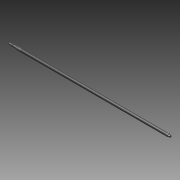
# Autodesk Inventor part: BNT 2010-2.61000-J1K Shaft
Saved by Autodesk Inventor 2016 (Build 200138000, 138)
## iProperties
Category: PARTsolutions
Company: THK
Created: 2017-05-30
Part Number: BNT 2010-2.61000-J1K Shaft
Catalog Web Link: www.cadenas.de
Description: BNT Shaft-
Vendor: THK
Document SubType Name: Modeling
Designer: psAdmin
Manufacturer: THK
Mass: 354.556 g
Surface Area: 729.515 cm^2
Volume: 354.556 cm^3
Density: 1 g/cm^3
Material: Generic
Appearance: PSOLRGB-192-192-192
PSOL_IDENT_0: {$CADENAS_DATA\23d-libs\thk\fed_screw\ball_screw\ball_screw\standard_lead_rbs\bnt\bnt_shaft.prj},206
PSOL_IDENT_1: {VTYP=3D},{NB=BNT 2010-2.61000-J1K Shaft},{LINA=BNT 2010-2.61000-J1K Shaft},{NN=BNT Shaft},{DATE=16
PSOL_IDENT_2: .05.2017 06:09:49},{GEOMDATE=28.04.2017 11:55:02},{VERSION=},{LINEID=520},{LINESUBID=-1},{WBVAR=ST,F
PSOL_IDENT_3: S,SS}  {NB=BNT 2010-2.61000-J1K Shaft},{LINA=BNT 2010-2.61000-J1K Shaft},{KT=DUMMY},{MN=BNT 2010-2.6
PSOL_IDENT_4: },{ST=1000},{FS=-J1},{SS=K},{OL=1166},{EL=2092},{L=58},{R1=11.300},{R2=11.300},{T1=2.500},{T2=2.500}
PSOL_IDENT_5: ,{P3=16.000},{P4=16.000},{B3=14.300},{B4=14.300},{G2=4.000},{G3=1.150},{G4=1.150},{F3=10.150},{F4=10
PSOL_IDENT_6: .150},{A3=15.000},{A4=15.000},{G1=4.000},{S1=12.000},{S2=13.000},{A1=15.000},{A2=15.000},{B1=12.000}
PSOL_IDENT_7: ,{B2=12.000},{J1=16.000},{SD=20},{J2=16.000},{M1=15.000},{M2=15.000},{P11=1.000},{P2=1.000},{P1=2.50
PSOL_IDENT_8: 0},{FSX='','None','-H1','Type_H1','-H2','Type_H2','-H3','Type_H3','-J1','Type_J1','-J2','Type_J2','-
PSOL_IDENT_9: J3','Type_J3'},{E3=13},{E4=13},{F1=20},{E1=40},{N1=6},{H1=9},{F2=20},{E2=49},{N2=6},{H2=9},{STX=2034
PSOL_IDENT_10: },{FSX1=75},{SSX1=13},{VERMN=1},{VERK=1}
NN: BNT Shaft
NB: BNT 2010-2.61000-J1K Shaft
NBSYN: $MN.$ST.$FS.$SS. Shaft
LINA: BNT 2010-2.61000-J1K Shaft
MN: BNT 2010-2.6
ST: 1000
FS: Type_J1
SS: Type_K
EL: 2092
L: 58
R1: 11.300
R2: 11.300
T1: 2.500
T2: 2.500
P3: 16.000
P4: 16.000
B3: 14.300
B4: 14.300
G2: 4.000
G3: 1.150
G4: 1.150
F3: 10.150
F4: 10.150
A3: 15.000
A4: 15.000
G1: 4.000
S1: 12.000
S2: 13.000
A1: 15.000
A2: 15.000
B1: 12.000
B2: 12.000
J1: 16.000
SD: 20
J2: 16.000
M1: 15.000
M2: 15.000
P11: 1.000
P2: 1.000
P1: 2.500
FSX: '','None','-H1','Type_H1','-H2','Type_H2','-H3','Type_H3','-J1','Type_J1','-J2','Type_J2','-J3','Type_J3'
E3: 13
E4: 13
F1: 20
E1: 40
N1: 6
H1: 9
F2: 20
E2: 49
N2: 6
H2: 9
VERMN: 1
SUPPLIER: THK
ARTICLENO: BNT 2010-2.61000-J1K Shaft
BOMINFO: BNT 2010-2.61000-J1K Shaft
CREATOR: CADENAS GmbH
Title: BNT 2010-2.61000-J1K Shaft
Author: Cadenas PARTsolutions
Autodesk Inventor part; units mm, degrees
ref_plane "YZ Plane" through (0, 0, 0) normal (1, 0, 0) x (0, 1, 0)
ref_plane "XZ Plane" through (0, 0, 0) normal (0, 1, 0) x (-1, 0, 0)
ref_plane "XY Plane" through (0, 0, 0) normal (0, 0, 1) x (1, 0, 0)
sketch "Sketch_1" plane through (0, 0, 0) normal (0, 0, 1) x (1, 0, 0)
  line L0 (1068, 0) -> (10, 0)
  line L1 (10, 0) -> (10, 10)
  line L2 (10, 10) -> (1068, 10)
  line L3 (1068, 10) -> (1068, 0)
  line L4 (1068, 0) -> (10, 0)
  constraints: 10 end point
revolve "Revolution1" add sketch "Sketch_1" angle 360 about axis through (1068, 0, 0) along (1, 0, 0)
thread "Thread1" size "M20x2.5" class "6g" standard "ISO Metric profile" full length
sketch "Sketch_10" plane through (0, 0, 0) normal (0, 1, 0) x (-1, 0, 0)
  line L0 (-10, 0) -> (75, 0)
  line L1 (75, 0) -> (75, -5.3333)
  line L2 (75, -5.3333) -> (74.3333, -6)
  line L3 (74.3333, -6) -> (55, -6)
  line L4 (55, -6) -> (55, -6.8865)
  line L5 (55, -6.8865) -> (54.3865, -7.5)
  line L6 (54.3865, -7.5) -> (15, -7.5)
  line L7 (15, -7.5) -> (15, -9)
  line L8 (15, -9) -> (14, -10)
  line L9 (14, -10) -> (-9.8, -10)
  line L10 (-9.8, -10) -> (-9.8, -8)
  line L11 (-9.8, -8) -> (-10, -8)
  line L12 (-10, -8) -> (-10, 0)
  line L13 (-10, 0) -> (75, 0)
  constraints: 28 end point
revolve "Revolution2" add sketch "Sketch_10" angle 360 about axis through (10, 0, 0) along (1, 0, 0)
thread "Thread2" size "M15x1" class "6g" standard "ISO Metric profile" length 11.3865
sketch "Sketch_11" plane through (0, 0, 8) normal (0, 0, 1) x (1, 0, 0)
  line L0 (-9, -10) -> (0, -10)
  line L1 (0, -10) -> (0, 10)
  line L2 (0, 10) -> (-9, 10)
  line L3 (-9, 10) -> (-9, -10)
  constraints: 8 end point
extrude "Extrusion1" cut sketch "Sketch_11" along normal blind 4
sketch "Sketch_12" plane through (0, 0, -8) normal (0, 0, 1) x (1, 0, 0)
  line L0 (-9, -10) -> (0, -10)
  line L1 (0, -10) -> (0, 10)
  line L2 (0, 10) -> (-9, 10)
  line L3 (-9, 10) -> (-9, -10)
  constraints: 8 end point
extrude "Extrusion2" cut sketch "Sketch_12" against normal blind 4
sketch "Sketch_16" plane through (0, 0, 0) normal (0, 0, 1) x (1, 0, 0)
  line L0 (1091, 0) -> (1068, 0)
  line L1 (1068, 0) -> (1068, 8)
  line L2 (1068, 8) -> (1068.2, 8)
  line L3 (1068.2, 8) -> (1068.2, 10)
  line L4 (1068.2, 10) -> (1077, 10)
  line L5 (1077, 10) -> (1078, 9)
  line L6 (1078, 9) -> (1078, 7.5)
  line L7 (1078, 7.5) -> (1087, 7.5)
  line L8 (1087, 7.5) -> (1087, 7.15)
  line L9 (1087, 7.15) -> (1088.15, 7.15)
  line L10 (1088.15, 7.15) -> (1088.15, 7.5)
  line L11 (1088.15, 7.5) -> (1090.25, 7.5)
  line L12 (1090.25, 7.5) -> (1091, 6.75)
  line L13 (1091, 6.75) -> (1091, 0)
  line L14 (1091, 0) -> (1068, 0)
  constraints: 30 end point
revolve "Revolution3" add sketch "Sketch_16" angle 360 about axis through (1091, 0, 0) along (1, 0, 0)
ref_plane "FSS_XY" through (-15, 0, 0) normal (1, 0, 0) x (0, 0, -1)
ref_plane "FSS_YZ" through (-15, 0, 0) normal (0, 0, -1) x (0, 1, 0)
ref_plane "FSS_ZX" through (-15, 0, 0) normal (0, 1, 0) x (1, 0, 0)
ref_plane "SSS_XY" through (1078, 0, 0) normal (1, 0, 0) x (0, 0, -1)
ref_plane "SSS_YZ" through (1078, 0, 0) normal (0, 0, -1) x (0, 1, 0)
ref_plane "SSS_ZX" through (1078, 0, 0) normal (0, 1, 0) x (1, 0, 0)
ref_plane "bnt_s_1_XY" through (0, 0, 0) normal (-1, 0, 0) x (0, 0, -1)
ref_plane "bnt_s_1_YZ" through (0, 0, 0) normal (0, 0, -1) x (0, -1, 0)
ref_plane "bnt_s_1_ZX" through (0, 0, 0) normal (0, -1, 0) x (-1, 0, 0)
body "Solid1"
